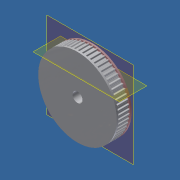
# Autodesk Inventor part: Synchrone Riemenscheibe T2.5 - Z60
Saved by Autodesk Inventor 2016 (Build 200138000, 138)
## iProperties
Created: 2015-09-10
Part Number: Synchrone Riemenscheibe T2.5 - Z60
Material: ABS-Kunststoff
Document SubType Name: Modeling
Designer: 4ndreas
Density: 1.06 g/cm^3
Appearance: Glatt - weiß
Mass: 19.2237 g
Surface Area: 62.0213 cm^2
Volume: 18.1356 cm^3
CustomPartVersion: 1
Author: 4ndreas
Autodesk Inventor part; units mm, degrees
ref_plane "YZ Plane" through (0, 0, 0) normal (1, 0, 0) x (0, 1, 0)
ref_plane "XZ Plane" through (0, 0, 0) normal (0, 1, 0) x (-1, 0, 0)
ref_plane "XY Plane" through (0, 0, 0) normal (0, 0, 1) x (1, 0, 0)
sketch "Riemenscheibenskizze" plane through (0, 0, 0) normal (0, 0, 1) x (1, 0, 0)
  circle A0 centre (0, 0) radius 23.8732 construction
  circle A1 centre (0, 0) radius 23.5732
  circle A2 centre (0, 0) radius 22.8232
  line L0 (-0.8673, 23.5573) -> (-0.525, 22.8232)
  line L1 (-0.525, 22.8232) -> (0.525, 22.8232)
  line L2 (0.525, 22.8232) -> (0.8673, 23.5573)
  line L3 (0, 0) -> (0, 23.5732) construction
  point P0 (0, 22.8232)
  dimension "d0" = 47.7465
  dimension "d1" = 0.3
  dimension "d2" = 0.75
  dimension "d3" = 50
  dimension "d4" = 1.05
  constraints: 8 end point, 3 coincident, 3 point on circle, 2 centre point, 1 horizontal, 1 midpoint, 1 point on line, 1 vertical, 1 vertical alignment, 3 other
  measures "d0" diameter of A0
  measures "d1" radial gap between concentric circles of A0 A1
  measures "d3" angle of L2 L0
  measures "d4" distance of L0.end L1.end
extrude "Grundkörper" add sketch "Riemenscheibenskizze" along normal mid plane 9 contours A2 | A1 L0 L1 L2 | L2 L1 L0 A1
extrude "Zahn" cut sketch "Riemenscheibenskizze" along normal through all both and the other way through all contours L2 L1 L0 A1 picked at (0, 23.322)
fillet "Fillet" radius 0.2 2 edges at (0.525, 22.8232, 0) (-0.525, 22.8232, 0)
fillet "Fillet" radius 0.3 4 edges at (-0.8673, 23.5573, 2.25) (-0.8673, 23.5573, -2.25) (0.8673, 23.5573, 2.25) (0.8673, 23.5573, -2.25)
pattern_circular "Zähne" count 60 over 360 about axis through (0, 0, -10) along (0, 0, 1) of "Zahn", "Fillet"
feature "Flansch links" [suppressed]
feature "Flansch rechts" [suppressed]
sketch "Skizze2" plane through (0, 0, 4.5) normal (0, 0, 1) x (1, 0, 0)
  circle A0 centre (0, 0) radius 23.5732
  arc A1 (1.3991, 23.5317) -> (1.0683, 23.549) centre (0, 0) ccw construction
  constraints: 1 centre point, 1 coincident, 1 concentric
extrude "Extrusion3" add sketch "Skizze2" against normal blind 1
sketch "Skizze3" plane through (0, 0, -4.5) normal (0, 0, -1) x (-1, 0, 0)
  circle A0 centre (0, 0) radius 23.5732 projected
extrude "Extrusion4" add sketch "Skizze3" against normal blind 1
sketch "Skizze4" plane through (0, 0, -4.5) normal (0, 0, -1) x (-1, 0, 0)
  circle A0 centre (0, 0) radius 15
  dimension "d21" = 30
  constraints: 1 centre point, 1 coincident
  measures "d21" diameter of A0
extrude "Extrusion5" add sketch "Skizze4" along normal blind 5
sketch "Skizze5" plane through (0, 0, -9.5) normal (0, 0, -1) x (-1, 0, 0)
  point P0 (0, 0)
hole "Bohrung1" at (0, 0, -9.5) direction (0, 0, 1) diameter 6 end through all
sketch "Skizze6" plane through (0, 0, -9.5) normal (0, 0, -1) x (-1, 0, 0)
  circle A0 centre (0, 0) radius 3 projected
  circle A1 centre (0, 0) radius 15 projected
  circle A2 centre (0, 0) radius 5
  dimension "d31" = 10
  constraints: 1 centre point, 1 coincident
  measures "d31" diameter of A2
extrude "Extrusion6" add sketch "Skizze6" along normal blind 1 contours A2
chamfer "Fase1" distance 1 angle 45 1 edges at (5, 0, -9.5)
sketch "Skizze7" plane through (0, 0, -9.5) normal (0, 0, -1) x (-1, 0, 0)
  line L0 (2.5, 11) -> (-2.5, 11)
  line L1 (-2.5, 11) -> (-2.5, 6)
  line L2 (-2.5, 6) -> (2.5, 6)
  line L3 (2.5, 6) -> (2.5, 11)
  circle A0 centre (0, 0) radius 6 projected
  circle A1 centre (0, 0) radius 3 projected
  circle A2 centre (0, 0) radius 15 projected
  line L4 (0, 0) -> (0, 15)
  dimension "d37" = 5
  dimension "d38" = 5
  constraints: 10 end point, 2 parallel, 1 horizontal, 1 perpendicular, 1 tangent, 1 vertical, 1 vertical alignment, 2 other
  measures "d37" distance between parallel lines of L1 L3
  measures "d38" distance between parallel lines of L2 L0
ref_plane "Arbeitsebene1" through (-2.5, 11, -9.5) normal (0, 1, 0) x (1, 0, 0)
sketch "Skizze8" plane through (-2.5, 11, -9.5) normal (0, 1, 0) x (1, 0, 0)
  line L0 (-17.5279, -6) -> (-18.02, -6) projected
  line L1 (-18.02, -6) -> (-18.02, -13) projected
  line L2 (-18.02, -13) -> (-17.5279, -13) projected
  line L3 (-17.5279, -13) -> (-17.5279, -6) projected
  line L4 (22.5279, -13) -> (23.02, -13) projected
  line L5 (23.02, -13) -> (23.02, -6) projected
  line L6 (23.02, -6) -> (22.5279, -6) projected
  line L7 (22.5279, -6) -> (22.5279, -13) projected
  line L8 (23.2433, -13) -> (23.3494, -13) projected
  line L9 (23.3494, -13) -> (23.3494, -14) projected
  line L10 (23.3494, -14) -> (-18.3494, -14) projected
  line L11 (-18.3494, -14) -> (-18.3494, -13) projected
  line L12 (-18.3494, -13) -> (-18.2433, -13) projected
  line L13 (-18.2433, -13) -> (-18.2433, -6) projected
  line L14 (-18.2433, -6) -> (-18.3494, -6) projected
  line L15 (-18.3494, -6) -> (-18.3494, -5) projected
  line L16 (-18.3494, -5) -> (-7.698, -5) projected
  line L17 (-7.698, -5) -> (-7.698, 0) projected
  line L18 (-7.698, 0) -> (12.698, 0) projected
  line L19 (12.698, 0) -> (12.698, -5) projected
  line L20 (12.698, -5) -> (23.3494, -5) projected
  line L21 (23.3494, -5) -> (23.3494, -6) projected
  line L22 (23.3494, -6) -> (23.2433, -6) projected
  line L23 (23.2433, -6) -> (23.2433, -13) projected
  line L24 (-12.5, -5) -> (17.5, -5) projected
  line L25 (-21.0732, -5) -> (26.0732, -5) projected
  line L26 (-0.5, -14) -> (-0.5, 1) projected
  line L27 (5.5, -14) -> (5.5, 1) projected
  line L28 (2.5, 0) -> (2.5, -6.5)
  circle A0 centre (2.5, -3.5) radius 1.5
  line L29 (5, -4.9434) -> (2.5, -6.3868)
  line L30 (2.5, -6.3868) -> (0, -4.9434)
  line L31 (0, -4.9434) -> (0, -2.0566)
  line L32 (0, -2.0566) -> (2.5, -0.6132)
  line L33 (2.5, -0.6132) -> (5, -2.0566)
  line L34 (5, -2.0566) -> (5, -4.9434)
  line L35 (-0.5, -6.3868) -> (5.5, -6.3868)
  point P0 (2.5, -9.5)
  point P1 (2.5, 0)
  dimension "d40" = 3
  dimension "d41" = 5
  constraints: 16 end point, 4 point on line, 2 perpendicular, 1 centre point, 1 coincident, 1 midpoint, 1 tangent, 13 other
  measures "d40" diameter of A0
  measures "d41" distance between parallel lines of L31 L34
ref_plane "Arbeitsebene2" through (-3, 11, -3.1132) normal (0, 0, -1) x (1, 0, 0)
extrude "Extrusion7" cut sketch "Skizze8" along normal through all both and the other way through all contours A0 L28 | L28 A0
extrude "Extrusion8" cut sketch "Skizze7" against normal up to surface (6.3868 mm away) contours L3 L2 L4 L0 | L4 L2 L1 L0
sketch "Skizze9" plane through (0, 0, -9.5) normal (0, 0, -1) x (-1, 0, 0)
  circle A0 centre (0, 0) radius 6 projected
  circle A1 centre (0, 0) radius 15 projected
  line L0 (11, 0) -> (-11, 0) construction
  line L1 (0, 6) -> (-2.5, 6) projected
  line L2 (-2.5, 6) -> (-2.5, 11) projected
  line L3 (-2.5, 11) -> (2.5, 11) projected
  line L4 (2.5, 11) -> (2.5, 6) projected
  line L5 (2.5, 6) -> (0, 6) projected
  dimension "d47" = 22
  constraints: 2 end point, 1 coincident, 1 midpoint, 1 vertical alignment
  measures "d47" distance of L0.start L0.end
hole "Bohrung2" [suppressed]
sketch "Skizze10" plane through (0, 0, 4.5) normal (0, 0, 1) x (1, 0, 0)
  circle A0 centre (0, 0) radius 3 projected
  circle A1 centre (0, 0) radius 23.5732 projected
  line L0 (-11, 3.1754) -> (-8.25, 1.5877)
  line L1 (-8.25, 1.5877) -> (-8.25, -1.5877)
  line L2 (-8.25, -1.5877) -> (-11, -3.1754)
  line L3 (-11, -3.1754) -> (-13.75, -1.5877)
  line L4 (-13.75, -1.5877) -> (-13.75, 1.5877)
  line L5 (-13.75, 1.5877) -> (-11, 3.1754)
  line L6 (11, 3.1754) -> (13.75, 1.5877)
  line L7 (13.75, 1.5877) -> (13.75, -1.5877)
  line L8 (13.75, -1.5877) -> (11, -3.1754)
  line L9 (11, -3.1754) -> (8.25, -1.5877)
  line L10 (8.25, -1.5877) -> (8.25, 1.5877)
  line L11 (8.25, 1.5877) -> (11, 3.1754)
  point P0 (-11, 0)
  point P1 (11, 0)
  point P2 (13.75, 0)
  dimension "d55" = 5.5
  constraints: 24 end point, 2 parallel, 1 midpoint, 1 vertical, 26 other
  measures "d55" distance between parallel lines of L4 L1
extrude "Extrusion9" [suppressed]
sketch "Skizze11" plane through (0, 0, 1.5) normal (0, 0, 1) x (1, 0, 0)
  circle A0 centre (-11, 0) radius 1.5 projected
  circle A1 centre (11, 0) radius 1.5 projected
  point P0 (0, 0)
extrude "Extrusion10" [suppressed]
chamfer "Fase2" distance 1 angle 45 1 edges at (15, 0, -9.5)
equation "\"d1\" = da_a"
equation "\"d2\" = da_hg"
equation "\"d3\" = 2 * da_fi"
equation "\"d4\" = da_bw"
equation "\"d7\" = da_bf"
equation "\"d9\" = da_rb"
equation "\"d10\" = da_rt"
equation "\"da_pb\" = 2.5"
equation "\"da_fi\" = 25deg"
equation "\"da_hg\" = 0.75"
equation "\"da_bw\" = 1.05"
equation "\"da_rb\" = 0.2"
equation "\"da_rt\" = 0.3"
equation "\"da_a\" = 0.3"
equation "\"da_bf\" = 10"
equation "\"da_wf\" = 0.8"
equation "\"da_hf\" = 0.8"
body "Solid1"
